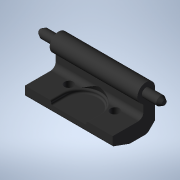
# Autodesk Inventor part: 1301.000_4_(1)
Saved by Autodesk Inventor 2021 (Build 250183000, 183)
## iProperties
Created: 2025-05-02
Part Number: 1301.000_4_(1)
Material: Generic
Catalog Web Link: www.cadenas.de
Description: Scharnier KX EB Edelstahl-Scharnier KX EB Edelstahl
Vendor: RITTAL
Document SubType Name: Modeling
Designer: psAdmin
Manufacturer: RITTAL
Mass: 1.84529 g
Surface Area: 14.2914 cm^2
Volume: 1.84529 cm^3
Density: 1 g/cm^3
Appearance: PSOLRGB-175-175-175
Category: PARTsolutions
Company: RITTAL
Title: 1301.000_4
Author: Cadenas PARTsolutions
Comments: Scharnier KX EB Edelstahl
PSOL_IDENT_0: {$CADENAS_DATA/23d-libs/rittal/schaltschranksys/edelstahl/kleingehause/parts_eb_edel_2_0/scharnier_k
PSOL_IDENT_1: x_eb_edel_new.prj},196 {VTYP=3D},{NB=1301.000_4_(1)},{LINA=1301.000_4},{NN=Scharnier KX EB Edelstahl
PSOL_IDENT_2: },{DATE=28.04.2025 21:10:48},{GEOMDATE=11.04.2025 11:21:29},{VERSION=},{LINEID=610},{WBVAR=DETAIL},{
PSOL_IDENT_3: WBNUMERIC=DETAIL}  {NB=1301.000_4_(1)},{LINA=1301.000_4},{KT=DUMMY},{BEST=1301.000},{DETAIL=1},{GEW=
PSOL_IDENT_4: 3,889},{CNSETIM80=EC000261},{CNSETIM90=EC000261},{CNSECLASS60=27-18-01-01},{CNSECLASS80=27-18-01-01}
PSOL_IDENT_5: ,{UNSPSC=31-26-15-02}
NB: 1301.000_4_(1)
NN: Scharnier KX EB Edelstahl
NT: Scharnier KX EB Edelstahl
NBSYN: $BEST._4_($DETAIL.)
LINA: 1301.000_4
CATALOG: Rittal
BEST: 1301.000
DETAIL: hoch
GEW: 3,889
CNSETIM80: EC000261
CNSETIM90: EC000261
CNSECLASS60: 27-18-01-01
CNSECLASS80: 27-18-01-01
UNSPSC: 31-26-15-02
SUPPLIER: RITTAL
ARTICLENO: 1301.000_4_(1)
BOMINFO: 1301.000_4
CREATOR: CADENAS GmbH
Autodesk Inventor part; units mm, degrees
sketch "Sketch_1" plane through (0, 0, 0) normal (1, 0, 0) x (0, 0, -1)
  line L0 (-6.5, 4.25) -> (-6.5, 2.0679)
  arc A0 (-6.5, 2.0679) -> (-6.2039, 1.645) centre (-6.05, 2.0679) ccw
  line L1 (-6.2039, 1.645) -> (-1.9329, 0.0905)
  arc A1 (-1.9329, 0.0905) -> (-1.4198, 0) centre (-1.4198, 1.5) ccw
  line L2 (-1.4198, 0) -> (2.6944, 0)
  arc A2 (2.6944, 0) -> (3.755, 0.4393) centre (2.6944, 1.5) ccw
  line L3 (3.755, 0.4393) -> (5.5, 2.1843)
  line L4 (5.5, 2.1843) -> (5.5, 10.25)
  arc A3 (5.5, 10.25) -> (1.9407, 7.9855) centre (3, 10.25) ccw
  arc A4 (2.2, 7.5779) -> (1.9407, 7.9855) centre (1.75, 7.5779) ccw
  line L5 (2.2, 7.5779) -> (2.2, 5.75)
  arc A5 (0.7, 4.25) -> (2.2, 5.75) centre (0.7, 5.75) ccw
  line L6 (0.7, 4.25) -> (-6.5, 4.25)
  constraints: 14 end point, 12 point on circle, 6 centre point
extrude "Extrusion1" add sketch "Sketch_1" along normal mid plane 24.8
sketch "Sketch2" plane through (-12.4, 0, -2.6944) normal (0, -1, 0) x (1, 0, 0)
  point P0 (18.9, 2.6944)
hole "Hole1" at (6.5, 0, 0) direction (0, 1, 0) diameter 2.459 depth 5.75
sketch "Sketch3" plane through (-12.4, 0, -2.6944) normal (0, -1, 0) x (1, 0, 0)
  point P0 (5.9, 2.6944)
hole "Hole2" at (-6.5, 0, 0) direction (0, 1, 0) diameter 2.459 depth 5.75
sketch "Sketch_5" plane through (0, 0, 6.5) normal (0, 0, 1) x (1, 0, 0)
  arc A0 (-5, 3.8) -> (-5.45, 4.25) centre (-5.45, 3.8) ccw
  line L0 (-5, 3.8) -> (-5, 3.7)
  arc A1 (-5, 3.7) -> (-4.55, 3.25) centre (-4.55, 3.7) ccw
  line L1 (-4.55, 3.25) -> (4.55, 3.25)
  arc A2 (4.55, 3.25) -> (5, 3.7) centre (4.55, 3.7) ccw
  line L2 (5, 3.7) -> (5, 3.8)
  arc A3 (5.45, 4.25) -> (5, 3.8) centre (5.45, 3.8) ccw
  line L3 (5.45, 4.25) -> (5.45, 7.25)
  line L4 (5.45, 7.25) -> (-5.45, 7.25)
  line L5 (-5.45, 7.25) -> (-5.45, 4.25)
  constraints: 12 end point, 8 point on circle, 4 centre point
extrude "Extrusion2" cut sketch "Sketch_5" against normal blind 3.7
sketch "Sketch_6" plane through (0, 0, 2.8) normal (0, 0, 1) x (1, 0, 0)
  line L0 (0, 3.25) -> (0, 7.25)
  line L1 (0, 7.25) -> (4.55, 7.25)
  line L2 (4.55, 7.25) -> (5.45, 4.25)
  arc A0 (5.45, 4.25) -> (5, 3.8) centre (5.45, 3.8) ccw
  line L3 (5, 3.8) -> (5, 3.7)
  arc A1 (4.55, 3.25) -> (5, 3.7) centre (4.55, 3.7) ccw
  line L4 (4.55, 3.25) -> (0, 3.25)
  line L5 (0, 3.25) -> (0, 7.25)
  constraints: 12 end point, 4 point on circle, 2 centre point
revolve "Revolution1" cut sketch "Sketch_6" angle 180 about axis through (0, 3.25, 2.8) along (0, 1, 0)
sketch "Sketch_8" plane through (0, 0, -3) normal (0, 0, 1) x (1, 0, 0)
  line L0 (17.5, 10.25) -> (-17.5, 10.25)
  line L1 (-17.5, 10.25) -> (-17.5, 10.925)
  line L2 (-17.5, 10.925) -> (-16.5, 11.5)
  line L3 (-16.5, 11.5) -> (16.5, 11.5)
  line L4 (16.5, 11.5) -> (17.5, 10.925)
  line L5 (17.5, 10.925) -> (17.5, 10.25)
  line L6 (17.5, 10.25) -> (-17.5, 10.25)
  constraints: 14 end point
revolve "Revolution2" add sketch "Sketch_8" angle 360 about axis through (17.5, 10.25, -3) along (1, 0, 0)
ref_plane "DECKEL_XY" through (0, 10.25, -3) normal (1, 0, 0) x (0, 0, -1)
ref_plane "DECKEL_YZ" through (0, 10.25, -3) normal (0, 0, -1) x (0, 1, 0)
ref_plane "DECKEL_ZX" through (0, 10.25, -3) normal (0, 1, 0) x (1, 0, 0)
ref_plane "HINGE_XY" through (0, 0, 0) normal (1, 0, 0) x (0, 0, -1)
ref_plane "HINGE_YZ" through (0, 0, 0) normal (0, 0, -1) x (0, 1, 0)
ref_plane "HINGE_ZX" through (0, 0, 0) normal (0, 1, 0) x (1, 0, 0)
body "Solid1"
